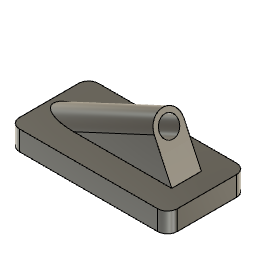
Standard Drawing Views - Practice (Autodesk Fusion 360 design; units mm, degrees)
Autodesk Fusion 360 part; units mm, degrees
sketch "Sketch1" plane through (0, 0, 0) normal (0, 1, 0) x (1, 0, 0)
  line L0 (50.8, 6.35) -> (-50.8, 6.35)
  line L1 (-50.8, 6.35) -> (-50.8, -6.35)
  line L2 (-50.8, -6.35) -> (50.8, -6.35)
  line L3 (50.8, -6.35) -> (50.8, 6.35)
  line L4 (50.8, 6.35) -> (-50.8, -6.35) construction
  line L5 (-50.8, 6.35) -> (50.8, -6.35) construction
  dimension "d1" = 101.6
  dimension "d2" = 12.7
  constraint horizontal L0
  constraint perpendicular L0 L1
  constraint parallel L0 L2
  constraint parallel L1 L3
  constraint coincident L4 origin
  constraint coincident L5 origin
  measures "d1" distance of L1.end L2.end
  measures "d2" distance of L0.end L1.end
extrude "Extrude1" add sketch "Sketch1" along normal mid plane 50.8
sketch "Sketch2" plane through (0, 0, 0) normal (0, 1, 0) x (1, 0, 0)
  line L0 (50.8, -6.35) -> (-50.8, -6.35)
  line L1 (-25.4, -6.35) -> (26.3955, -30.5026)
  dimension "d5" = 25.4
  dimension "d6" = 25
  dimension "d7" = 57.15
  constraint coincident L0 L1.start
  measures "d5" horizontal distance of origin L1.start
  measures "d6" angle of L0 L1
  measures "d7" distance of L1.start L1.end
ref_plane "WorkPlane1" through (26.3955, 0, 30.5026) normal (0.906308, 0, 0.422618) x (0, 1, 0)
sketch "Sketch3" plane through (26.3955, 0, 30.5026) normal (0.906308, 0, 0.422618) x (0, 1, 0)
  circle A0 centre (0, 0) radius 6.35
  circle A1 centre (0, 0) radius 9.525
  line L0 (-9.525, 0) -> (-9.525, -26.6495)
  line L1 (-9.525, -26.6495) -> (9.525, -26.6495)
  line L2 (9.525, -26.6495) -> (9.525, 0)
  line L3 (25.4, -26.6495) -> (-25.4, -26.6495)
  dimension "d9" = 12.7
  dimension "d10" = 19.05
  constraint coincident A0.centre A1.centre
  constraint concentric A0 A1
  constraint coincident A1 L0.start
  constraint vertical L0
  constraint perpendicular L0 L1
  constraint coincident A1 L2.end
  constraint tangent A1 L2
  constraint vertical L2
  constraint tangent A1 L0
  constraint collinear L1 L3
  measures "d9" diameter of A0
  measures "d10" diameter of A1
extrude "Extrude2" add sketch "Sketch3" along normal up to surface contours A0 | A1 | A1 L0 L1 L2 L3 end surface through (-50.8, 0, 6.35) normal (0, 0, 1) offset 0
extrude "Extrude3" cut sketch "Sketch3" against normal blind 25.4 contours A0
fillet "Fillet1" radius 6.35 4 edges at (-50.8, -25.4, 0) (-50.8, 25.4, 0) (50.8, 25.4, 0) (50.8, -25.4, 0)
